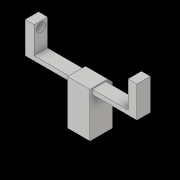
# Autodesk Inventor part: TubePostV1
Saved by Autodesk Inventor 2019 (Build 230136000, 136)
## iProperties
Created: 2021-09-17
Part Number: TubePostV1
Material: Generic
Document SubType Name: Modeling
Designer: timmy
Density: 1 g/cm^3
Appearance: Default
Author: timmy
Autodesk Inventor part; units mm, degrees
ref_plane "YZ Plane" through (0, 0, 0) normal (1, 0, 0) x (0, 1, 0)
ref_plane "XZ Plane" through (0, 0, 0) normal (0, 1, 0) x (-1, 0, 0)
ref_plane "XY Plane" through (0, 0, 0) normal (0, 0, 1) x (1, 0, 0)
sketch "Sketch1" plane through (0, 0, 0) normal (0, 1, 0) x (-1, 0, 0)
  line L0 (0, 0) -> (127, 0)
  line L1 (127, 0) -> (127, -127)
  line L2 (127, -127) -> (0, -127)
  line L3 (0, -127) -> (0, 0)
  dimension "d0" = 127
  dimension "d1" = 127
  constraints: 8 end point, 2 parallel, 1 horizontal, 1 perpendicular
  measures "d0" distance of L1.end L2.end
  measures "d1" distance of L0.end L1.end
extrude "Extrusion1" add sketch "Sketch1" along normal blind 254
sketch "Sketch3" plane through (0, 0, 0) normal (0, -1, 0) x (1, 0, 0)
  line L0 (0, -127) -> (-127, -127) projected
  line L1 (-127, -127) -> (-127, 0) projected
  line L2 (0, 0) -> (0, -127) projected
  line L3 (-127, 0) -> (0, 0) projected
  circle A0 centre (-31.75, -31.75) radius 6.35
  circle A1 centre (-95.25, -31.75) radius 6.35
  circle A2 centre (-95.25, -95.25) radius 6.35
  circle A3 centre (-31.75, -95.25) radius 6.35
  dimension "d5" = 12.7
  dimension "d6" = 12.7
  dimension "d7" = 12.7
  dimension "d8" = 12.7
  constraints: 4 centre point
  measures "d5" diameter of A0
  measures "d6" diameter of A1
  measures "d7" diameter of A2
  measures "d8" diameter of A3
extrude "Extrusion2" add sketch "Sketch3" along normal blind 25.4 contours A0 | A1 | A2 | A3
thread "Thread1" size "1/2-13 UNC" class "2A" standard "ANSI Unified Screw Threads" full length
thread "Thread2" size "1/2-13 UNC" class "2A" standard "ANSI Unified Screw Threads" full length
thread "Thread3" size "1/2-13 UNC" class "2A" standard "ANSI Unified Screw Threads" full length
thread "Thread4" size "1/2-13 UNC" class "2A" standard "ANSI Unified Screw Threads" full length
chamfer "Chamfer1" distance 25.4 angle 45 1 edges at (-63.5, 254, -127)
sketch "Sketch5" plane through (0, 0, 0) normal (1, 0, 0) x (0, 0, -1)
  line L0 (127, 0) -> (127, 228.6) projected
  line L1 (101.6, 254) -> (0, 254) projected
  line L2 (12.7, 223.2608) -> (88.9, 223.2608)
  line L3 (88.9, 223.2608) -> (88.9, 248.6608)
  line L4 (88.9, 248.6608) -> (12.7, 248.6608)
  line L5 (12.7, 248.6608) -> (12.7, 223.2608)
  line L6 (12.7, 223.2608) -> (88.9, 248.6608) construction
  line L7 (88.9, 223.2608) -> (12.7, 248.6608) construction
  point P0 (0, 0)
  point P1 (50.8, 235.9608)
  dimension "d22" = 76.2
  dimension "d23" = 25.4
  constraints: 12 end point, 2 midpoint, 2 parallel, 1 horizontal, 1 perpendicular
  measures "d22" distance of L4.end L3.end
  measures "d23" distance of L3.end L2.end
extrude "Extrusion3" add sketch "Sketch5" along normal blind 254
sketch "Sketch6" plane through (0, 248.6608, -12.7) normal (0, 1, 0) x (1, 0, 0)
  line L0 (0, 0) -> (254, 0) projected
  line L1 (254, 0) -> (203.2, 0)
  line L2 (203.2, 0) -> (203.2, 76.2)
  line L3 (203.2, 76.2) -> (254, 76.2)
  line L4 (254, 76.2) -> (254, 0)
  point P0 (0, -12.7)
  dimension "d26" = 50.8
  dimension "d27" = 76.2
  constraints: 8 end point, 2 parallel, 1 horizontal, 1 perpendicular
  measures "d26" distance of L2.end L3.end
  measures "d27" distance of L1.end L2.end
extrude "Extrusion4" add sketch "Sketch6" along normal blind 152.4
sketch "Sketch7" plane through (203.2, 248.6608, -88.9) normal (-1, 0, 0) x (0, 0, 1)
  line L0 (0, 152.4) -> (76.2, 152.4) projected
  line L1 (38.1, 152.4) -> (38.1, 120.65)
  circle A0 centre (38.1, 120.65) radius 25.4
  point P0 (88.9, -248.6608)
  dimension "d30" = 31.75
  dimension "d31" = 50.8
  constraints: 2 end point, 1 centre point, 1 coincident, 1 midpoint, 1 vertical
  measures "d30" distance of L1.start L1.end
  measures "d31" diameter of A0
extrude "Extrusion5" cut sketch "Sketch7" against normal blind 38.1
sketch "Sketch8" plane through (-127, 0, -127) normal (-1, 0, 0) x (0, 0, 1)
  line L0 (114.3, 223.2608) -> (114.3, 248.6608) projected
  line L1 (114.3, 248.6608) -> (38.1, 248.6608) projected
  line L2 (38.1, 223.2608) -> (114.3, 223.2608) projected
  line L3 (114.3, 223.2608) -> (114.3, 248.6608) projected
  line L4 (114.3, 248.6608) -> (38.1, 248.6608) projected
  line L5 (38.1, 248.6608) -> (38.1, 223.2608) projected
  line L6 (38.1, 223.2608) -> (114.3, 223.2608) projected
  line L7 (25.4, 254) -> (0, 228.6) projected
  line L8 (127, 254) -> (25.4, 254) projected
  line L9 (127, 0) -> (127, 254) projected
  line L10 (0, 0) -> (127, 0) projected
  line L11 (0, 0) -> (0, 228.6) projected
extrude "Extrusion6" add sketch "Sketch8" along normal blind 254 contours L2 L5 L1 L0
sketch "Sketch9" plane through (-127, 248.6608, -12.7) normal (0, 1, 0) x (1, 0, 0)
  line L0 (0, 76.2) -> (0, 0) projected
  line L1 (0, 76.2) -> (-254, 76.2) projected
  line L2 (-254, 0) -> (-254, 76.2) projected
  line L3 (0, 0) -> (-254, 0) projected
  line L4 (-254, 76.2) -> (-254, 0) projected
  line L5 (-254, 0) -> (-203.2, 0)
  line L6 (-203.2, 0) -> (-203.2, 76.2)
  line L7 (-203.2, 76.2) -> (-254, 76.2)
  line L8 (-254, 76.2) -> (-254, 0)
  point P0 (127, -12.7)
  dimension "d36" = 50.8
  dimension "d37" = 76.2
  constraints: 8 end point, 2 parallel, 1 horizontal, 1 perpendicular
  measures "d36" distance of L7.end L6.end
  measures "d37" distance of L6.end L5.end
extrude "Extrusion7" add sketch "Sketch9" along normal blind 152.4 contours L6 L3 L2 L1
sketch "Sketch10" plane through (-330.2, 248.6608, -12.7) normal (1, 0, 0) x (0, 0, -1)
  circle A0 centre (38.1, 120.65) radius 25.4 projected
  circle A1 centre (38.1, 120.65) radius 25.4 projected
  point P0 (-12.7, -248.6608)
extrude "Extrusion8" cut sketch "Sketch10" against normal blind 38.1
body "Solid1"
